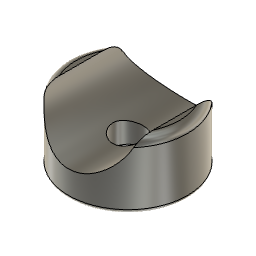
Saddles v3 (Autodesk Fusion 360 design; units mm, degrees)
Autodesk Fusion 360 part; units mm, degrees
sketch "Body1" plane through (0, 0, 0) normal (0, 1, 0) x (1, 0, 0)
  line L0 (-4, -15) -> (-4, 0)
  line L1 (-4, 0) -> (0, 0)
  line L2 (-15.5, 0) -> (-15.5, -5)
  line L3 (-4, -15) -> (-13.5, -15)
  line L4 (-15.5, -5) -> (-15.5, -13)
  arc A0 (-15.5, -13) -> (-13.5, -15) centre (-13.5, -13) ccw
  line L5 (-15.5, 0) -> (-4, 0)
  point P0 (-13.5, -13)
  point P1 (-13.5, -13)
  point P2 (-15.5, -5)
  point P3 (-15.5, 0)
  dimension "d188" = 4
  dimension "d190" = 13.5
  dimension "d191" = 15
  dimension "d216" = 5
  dimension "d218" = 13
  dimension "d219" = 4
  dimension "d284" = 15.5
  constraint vertical L0
  constraint coincident L1.end origin
  constraint perpendicular L0 L1
  constraint coincident P1 P0
  constraint coincident P2 L2.end
  constraint tangent L3 A0
  constraint tangent L4 A0
  constraint vertical L2
  constraint coincident P3 L2.start
  constraint perpendicular L0 L5
  measures "d188" distance of L1.end L0.end
  measures "d190" horizontal distance of L1.end P1
  measures "d191" distance of L0.end L0.start
  measures "d216" vertical distance of L1.end P2
  measures "d218" vertical distance of L1.end P1
  measures "d219" diameter of A0
  measures "d284" distance of L1.end P3
sketch "Tube1" plane through (0, 0, 0) normal (0, 1, 0) x (1, 0, 0)
  circle A0 centre (0, -17.5) radius 12.5
  point P0 (-4, -15)
  dimension "d200" = 17.5
  dimension "d201" = 25
  dimension "d202" = 4
  measures "d200" vertical distance of A0.centre origin
  measures "d201" diameter of A0
  measures "d202" horizontal distance of A0.centre P0
sketch "Body2" plane through (0, 0, 0) normal (0, 1, 0) x (1, 0, 0)
  line L0 (0, 0) -> (-4, 0)
  line L1 (-4, 0) -> (-4, 0.001)
  line L2 (0, 0) -> (-15.5, 0)
  line L3 (-4, 0.001) -> (-15.4997, 0.001)
  line L4 (-15.5, 0) -> (-15.5, 0.0007)
  arc A0 (-15.4997, 0.001) -> (-15.5, 0.0007) centre (-15.4997, 0.0007) ccw
  point P0 (-15.4997, 0.0007)
  dimension "d224" = 0.001
  dimension "d228" = 15.5
  dimension "d229" = 0.0005
  dimension "d267" = 4
  constraint coincident L0.start L2.start
  constraint horizontal L0
  constraint perpendicular L0 L1
  constraint parallel L0 L2
  constraint perpendicular L1 L3
  constraint coincident P0 A0.centre
  constraint tangent L3 A0
  constraint tangent L4 A0
  constraint perpendicular L2 L4
  measures "d224" distance of L0.end L1.end
  measures "d228" distance of L0.start L2.end
  measures "d229" diameter of A0
  measures "d267" distance of L0.start L0.end
sketch "Tube2" plane through (0, 0, 0) normal (0, 1, 0) x (1, 0, 0)
  line L0 (-12.5, 12.5) -> (12.5, 12.5)
  line L1 (0, 0) -> (0, 12.5)
  line L2 (0, 12.5) -> (23, 12.5)
  circle A0 centre (0, 12.5) radius 12.5
  dimension "d304" = 25
  dimension "d305" = 12.5
  dimension "d306" = 0
  constraint coincident L1.start origin
  constraint vertical L1
  constraint midpoint L0 L1.end
  constraint perpendicular L1 L2
  constraint coincident L0.start A0
  constraint coincident L1.start A0
  constraint coincident L0.end A0
  constraint horizontal L2
  measures "d304" distance of L0.start L0.end
  measures "d305" distance of L1.start L1.end
  measures "d306" angle of L0 L2
sketch "Flange" plane through (0, 0, 0) normal (0, 1, 0) x (1, 0, 0)
  line L0 (-12.75, 2) -> (-12.75, 0)
  line L1 (-4, 0) -> (-12.75, 0)
  line L2 (-4, 0) -> (0, 0)
  line L3 (-14.5, 2) -> (-12.75, 2)
  line L4 (-15.5, 1) -> (-15.5, 0)
  line L5 (-15.5, 0) -> (-12.75, 0)
  arc A0 (-14.5, 2) -> (-15.5, 1) centre (-14.5, 1) ccw
  line L6 (0, 0) -> (0, -5)
  point P0 (-13.5, -13)
  point P1 (-15.5, 2)
  point P2 (-13.5, -13)
  point P3 (0, -5)
  dimension "d268" = 4
  dimension "d271" = 12.75
  dimension "d273" = 15.5
  dimension "d278" = 1
  dimension "d281" = 5
  dimension "d282" = 5
  constraint coincident L2.end L6.start
  constraint perpendicular L0 L1
  constraint coincident P2 P0
  constraint perpendicular L0 L3
  constraint coincident P1 L3
  constraint perpendicular L0 L5
  constraint vertical L4
  constraint perpendicular L3 L4
  constraint tangent L4 A0
  constraint tangent L3 A0
  constraint coincident P3 L6.end
  constraint vertical L6
  constraint perpendicular L2 L6
  measures "d268" distance of L2.end L1.start
  measures "d271" distance of L2.end L0.end
  measures "d273" horizontal distance of L2.end P1
  measures "d278" radius of A0
  measures "d281" distance of L2.end P3
  measures "d282" distance of L2.end P3
revolve "Revolve24" add sketch "Body1" angle 360 about axis through (0, 0, 1.75) along (0, 0, 1)
extrude "Extrude19" cut sketch "Tube1" along normal mid plane 200
revolve "Revolve25" add sketch "Body2" angle 360 about axis through (0, 0, 5) along (0, 0, 1) contours L1 L2 L3 L4 A0
extrude "Extrude20" cut sketch "Tube2" along normal mid plane 200
revolve "Revolve26" add sketch "Flange" angle 360 about axis through (0, 0, 0) along (0, 0, -1)
sketch "Sketch6" plane through (0, 0, 0) normal (1, 0, 0) x (0, 1, 0)
  circle A0 centre (0, 17.5) radius 12.5
  dimension "d115" = 25
  dimension "d118" = 17.5
  measures "d115" diameter of A0
  measures "d118" distance of A0.centre origin
revolve "Revolve3" [suppressed]
extrude "Extrude5" [suppressed]
equation "boltHoleDiameter = 8 mm"
equation "d115 = diameterTube1"
equation "d118 = ( diameterTube1 / 2 ) + 5 mm"
equation "d134 = max(diameterTube1; diameterTube2)"
equation "saddleType = 1" comment "1 = T type, 2 = X type"
equation "diameterTube1 = 25 mm"
equation "diameterTube2 = 25 mm"
equation "crossAngle = 0 deg"
equation "bodyHeight = 5 mm"
equation "tube1BodyHeight = ( diameterTube1 / 2 ) - 2.5 mm"
equation "tube1BodyRadius = ( diameterTube1 / 2 ) + 3 mm"
equation "tube2BodyDiameter = ( diameterTube2 / 2 ) + 3 mm"
equation "tube2BodyHeight = if(saddleType == 1; 0.001 mm; ( diameterTube2 / 2 ) - 2.5 mm)"
equation "d188 = boltHoleDiameter / 2"
equation "d190 = tube1BodyRadius - 2 mm"
equation "d191 = tube1BodyHeight + bodyHeight"
equation "d200 = bodyHeight + ( diameterTube1 / 2 )"
equation "d201 = diameterTube1"
equation "d202 = boltHoleDiameter / 2"
equation "d216 = bodyHeight"
equation "d218 = tube1BodyHeight + bodyHeight - 2 mm"
equation "d224 = tube2BodyHeight"
equation "d228 = tube2BodyDiameter"
equation "d229 = ( if(saddleType == 1; 0.0005; 4) ) * 1 mm"
equation "d267 = boltHoleDiameter / 2"
equation "d268 = boltHoleDiameter / 2"
equation "d271 = ( diameterTube2 + 0.5 mm ) / 2"
equation "d273 = tube2BodyDiameter"
equation "d281 = bodyHeight"
equation "d282 = if(saddleType == 1; bodyHeight; 0.001 mm)"
equation "d284 = tube2BodyDiameter"
equation "d304 = diameterTube2"
equation "d305 = diameterTube2 / 2"
equation "d306 = crossAngle"
